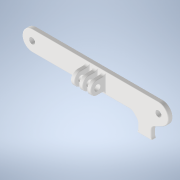
# Autodesk Inventor part: BackPlate
Saved by Autodesk Inventor 2021.3 (Build 253353010, 353A)
## iProperties
Created: 2021-08-11
Part Number: BackPlate
Material: Generisch
Document SubType Name: Modeling
Designer: Markus
Density: 1 g/cm^3
Appearance: Vorgabe
Author: Markus
Autodesk Inventor part; units mm, degrees
ref_plane "YZ Plane" through (0, 0, 0) normal (1, 0, 0) x (0, 1, 0)
ref_plane "XZ Plane" through (0, 0, 0) normal (0, 1, 0) x (-1, 0, 0)
ref_plane "XY Plane" through (0, 0, 0) normal (0, 0, 1) x (1, 0, 0)
sketch "Skizze2" plane through (0, 0, 0) normal (0, 0, 1) x (1, 0, 0)
  circle A0 centre (-47.5, 0) radius 2.408 projected
  spline S0 degree 3 poles (49.5, 0) (49.4999, -0.2484) (49.4548, -0.5089) (49.2125, -1.0889) (49.0309, -1.2975) (48.7582, -1.5703) (48.5453, -1.731) (48.0037, -1.9569) (47.7467, -1.9965) (47.2909, -2.0034) (47.0244, -1.964) (46.487, -1.7487) (46.2786, -1.598) (45.965, -1.3008) (45.7973, -1.0919) (45.5661, -0.5741) (45.5068, -0.3132) (45.4951, 0.1837) (45.5289, 0.4397) (45.7314, 0.9792) (45.8833, 1.1989) (46.2267, 1.567) (46.4444, 1.7165) (46.9007, 1.9251) (47.1526, 1.9859) (47.6719, 2.0102) (47.9359, 1.9699) (48.426, 1.7911) (48.6459, 1.6588) (49.0294, 1.3148) (49.1871, 1.1055) (49.4158, 0.6317) (49.483, 0.3718) (49.5059, -0.0571) (49.5014, -0.3263) (49.3091, -0.8923) (49.1761, -1.1223) (48.7992, -1.5514) (48.5744, -1.7005) (48.1516, -1.9082) (47.9012, -1.9759) (47.379, -2.0142) (47.1127, -1.9802) (46.6164, -1.8125) (46.3915, -1.6845) (45.9998, -1.3478) (45.8386, -1.1432) (45.5989, -0.6757) (45.5252, -0.4144) (45.4889, 0.0756) (45.5077, 0.3319) (45.6649, 0.8307) (45.7859, 1.0688) (46.1745, 1.5312) (46.4014, 1.6839) (46.8129, 1.8958) (47.0618, 1.9681) (47.6036, 2.0179) (47.8688, 1.9805) (48.3226, 1.8379) (48.5568, 1.7213) (48.9882, 1.3646) (49.1468, 1.159) (49.3855, 0.718) (49.4651, 0.4586) (49.5149, -0.0583) (49.4916, -0.3114) (49.3754, -0.7146) (49.2791, -0.9773) (48.883, -1.4729) (48.6723, -1.6385) (48.2327, -1.8787) (47.986, -1.9568) (47.4539, -2.0188) (47.1942, -1.9917) (46.756, -1.8682) (46.5093, -1.7643) (46.0388, -1.3961) (45.8712, -1.1849) (45.6506, -0.7906) (45.5549, -0.5486) (45.4775, 0.0404) (45.5118, 0.3057) (45.6296, 0.7488) (45.7375, 0.9855) (46.0612, 1.4125) (46.2535, 1.5852) (46.7029, 1.8534) (46.9543, 1.9423) (47.5294, 2.0243) (47.7984, 1.9884) (48.2415, 1.8743) (48.471, 1.7665) (48.9025, 1.4534) (49.0822, 1.2491) (49.3309, 0.8369) (49.4293, 0.5973) (49.5203, 0.0353) (49.5003, -0.2264) (49.3956, -0.6801) (49.2956, -0.9278) (48.9765, -1.373) (48.7884, -1.5513) (48.3813, -1.8093) (48.1346, -1.921) (47.5473, -2.0204) (47.2807, -2.0017) (46.7822, -1.8871) (46.5512, -1.7754) (46.1433, -1.4937) (45.9552, -1.2978) (45.6737, -0.8552) (45.5789, -0.6134) (45.4861, -0.1049) (45.4894, 0.1543) (45.5958, 0.6669) (45.7007, 0.9133) (45.9974, 1.3444) (46.1823, 1.5263) (46.5664, 1.7805) (46.8093, 1.9037) (47.3804, 2.0136) (47.6462, 2.0118) (48.2049, 1.8967) (48.4387, 1.7768) (48.8257, 1.5214) (49.0177, 1.3295) (49.3097, 0.8904) (49.4097, 0.6486) (49.5112, 0.143) (49.5131, -0.1147) (49.4169, -0.6302) (49.3158, -0.8803) (49.0266, -1.3169) (48.8451, -1.5021) (48.4436, -1.7786) (48.2042, -1.8945) (47.6624, -2.0105) (47.3974, -2.0146) (46.8418, -1.9125) (46.6055, -1.8006) (46.2068, -1.5487) (46.0132, -1.3634) (45.6983, -0.9137) (45.6, -0.6683) (45.4987, -0.2146) (45.4809, 0.0417) (45.5679, 0.5809) (45.6616, 0.8311) (45.9276, 1.2587) (46.0988, 1.4525) (46.371, 1.6523) (46.4267, 1.6889) (46.5266, 1.7478) (46.5702, 1.7715) (46.6733, 1.8225) (46.7334, 1.8484) (46.8365, 1.8872) (46.8793, 1.9017) (46.9444, 1.9214) (46.9664, 1.9276) (46.9994, 1.9364) (47.0105, 1.9392) (47.0324, 1.9446) (47.0411, 1.9467) (47.055, 1.9499) knots -7.965563 -7.965563 -7.965563 -7.965563 -7.879878 -7.879878 -7.775933 -7.775933 -7.637096 -7.637096 -7.502303 -7.502303 -7.353289 -7.353289 -7.204313 -7.204313 -7.050891 -7.050891 -6.916528 -6.916528 -6.799787 -6.799787 -6.676821 -6.676821 -6.527582 -6.527582 -6.372473 -6.372473 -6.211341 -6.211341 -6.055863 -6.055863 -5.89713 -5.89713 -5.736133 -5.736133 -5.636646 -5.636646 -5.558136 -5.558136 -5.466551 -5.466551 -5.357138 -5.357138 -5.243045 -5.243045 -5.13302 -5.13302 -5.022453 -5.022453 -4.908273 -4.908273 -4.812824 -4.812824 -4.73083 -4.73083 -4.639185 -4.639185 -4.524818 -4.524818 -4.396814 -4.396814 -4.272633 -4.272633 -4.150707 -4.150707 -4.012003 -4.012003 -3.882134 -3.882134 -3.795246 -3.795246 -3.723503 -3.723503 -3.647638 -3.647638 -3.565157 -3.565157 -3.495008 -3.495008 -3.42854 -3.42854 -3.368826 -3.368826 -3.306751 -3.306751 -3.236245 -3.236245 -3.17149 -3.17149 -3.104728 -3.104728 -3.025673 -3.025673 -2.930316 -2.930316 -2.823096 -2.823096 -2.726193 -2.726193 -2.627121 -2.627121 -2.525192 -2.525192 -2.435262 -2.435262 -2.35659 -2.35659 -2.281415 -2.281415 -2.193498 -2.193498 -2.090417 -2.090417 -1.990838 -1.990838 -1.891283 -1.891283 -1.788434 -1.788434 -1.689604 -1.689604 -1.611023 -1.611023 -1.545671 -1.545671 -1.469561 -1.469561 -1.365272 -1.365272 -1.263913 -1.263913 -1.163903 -1.163903 -1.059543 -1.059543 -0.959854 -0.959854 -0.869763 -0.869763 -0.788481 -0.788481 -0.695826 -0.695826 -0.576354 -0.576354 -0.448226 -0.448226 -0.325928 -0.325928 -0.209919 -0.209919 -0.105155 -0.105155 -0.079207 -0.079207 -0.060274 -0.060274 -0.03511 -0.03511 -0.017578 -0.017578 -0.008738 -0.008738 -0.004303 -0.004303 -0.000001 -0.000001 -0.000001 -0.000001 projected
  arc A1 (53.1427, -9.7735) -> (53.1427, 9.7735) centre (47.5, 0) ccw projected
  line L0 (-47.5, 0) -> (47.5, 0) construction
  circle A2 centre (-47.5, 0) radius 2.25
  circle A3 centre (47.5, 0) radius 2.25
  line L1 (42.01, -13.7) -> (42.01, -18)
  line L2 (42.01, -19) -> (32.01, -19)
  line L3 (32.01, -18) -> (32.01, -13.7)
  line L4 (32.29, -13.7) -> (41.73, -13.7) projected
  line L5 (45.2896, -14.5) -> (-45.2896, -14.5) projected
  line L6 (32.01, -19.5) -> (42.01, -19.5) construction
  line L7 (32.01, -20) -> (42.01, -20)
  line L8 (42.01, -19) -> (32.01, -19)
  arc A4 (31.61, -19.2) -> (32.01, -20) centre (32.01, -19.5) ccw
  arc A5 (42.01, -20) -> (42.41, -19.2) centre (42.01, -19.5) ccw
  arc A6 (42.01, -18) -> (42.41, -19.2) centre (44.01, -18) ccw
  arc A7 (31.61, -19.2) -> (32.01, -18) centre (30.01, -18) ccw
  arc A8 (32.01, -13.7) -> (30.8384, -10.8716) centre (28.01, -13.7) ccw
  arc A9 (44.1798, -10.1433) -> (42.01, -13.7) centre (46.01, -13.7) ccw
  arc A10 (-47.5, 7.5) -> (-47.5, -7.5) centre (-47.5, 0) ccw
  arc A11 (50.9317, -6.6688) -> (47.5, 7.5) centre (47.5, 0) ccw
  line L9 (-47.5, 7.5) -> (47.5, 7.5)
  line L10 (44.1798, -10.1433) -> (50.9317, -6.6688)
  line L11 (-47.5, -7.5) -> (25.81, -7.5)
  arc A12 (28.6384, -8.6716) -> (25.81, -7.5) centre (25.81, -11.5) ccw
  line L12 (28.6384, -8.6716) -> (30.8384, -10.8716)
  point P0 (0, 0)
  point P1 (0, 0)
  point P2 (37.01, -13.7)
  point P3 (37.01, -19)
  point P4 (37.01, -19.5)
  point P5 (37.01, -19)
  dimension "d3" = 4.5
  dimension "d4" = 4.5
  dimension "d28" = 10
  dimension "d29" = 4.5
  dimension "d30" = 1
  dimension "d48" = 2
  dimension "d49" = 4
  dimension "d54" = 15
  dimension "d55" = 4
  dimension "d59" = 135
  constraints: 26 end point, 20 point on circle, 19 tangent, 11 centre point, 6 vertical alignment, 5 midpoint, 4 horizontal, 4 point on line, 2 coincident, 2 concentric, 2 equal radius, 2 horizontal alignment, 2 parallel
  measures "d3" diameter of A2
  measures "d4" diameter of A3
  measures "d28" distance of L2.start L2.end
  measures "d29" distance between parallel lines of L5 L2
  measures "d30" distance between parallel lines of L7 L2
  measures "d48" radius of A6
  measures "d49" radius of A8
  measures "d54" distance between parallel lines of L9 L11
  measures "d55" radius of A12
  measures "d59" angle of L11 L12
extrude "Extrusion1" add sketch "Skizze2" along normal blind 3 contours A0 | L1 L5 L3 A8 L12 A12 L11 A10 L9 A11 L10 A9 | L1 A6 A5 L7 A4 A7 L3 L5
sketch "Skizze3" plane through (0, 0, 3) normal (0, 0, 1) x (1, 0, 0)
  line L0 (1.5, -5) -> (-1.5, -5)
  line L1 (-1.5, -5) -> (-1.5, 5)
  line L2 (-1.5, 5) -> (1.5, 5)
  line L3 (1.5, 5) -> (1.5, -5)
  line L4 (7.57, -5) -> (4.57, -5)
  line L5 (4.57, -5) -> (4.57, 5)
  line L6 (4.57, 5) -> (7.57, 5)
  line L7 (7.57, 5) -> (7.57, -5)
  line L8 (-4.57, -5) -> (-7.57, -5)
  line L9 (-7.57, -5) -> (-7.57, 5)
  line L10 (-7.57, 5) -> (-4.57, 5)
  line L11 (-4.57, 5) -> (-4.57, -5)
  point P0 (0, 0)
  point P1 (-1.5, 0)
  point P2 (0, -5)
  point P3 (6.07, -5)
  point P4 (4.57, 0)
  point P5 (-6.07, -5)
  point P6 (-7.57, 0)
  dimension "d7" = 10
  dimension "d8" = 3
  dimension "d11" = 6.07
  dimension "d18" = 6.07
  constraints: 24 end point, 3 horizontal, 2 collinear, 2 midpoint, 2 parallel, 1 horizontal alignment, 1 perpendicular, 1 vertical alignment, 18 other
  measures "d7" distance of L0.end L1.end
  measures "d8" distance of L1.end L2.end
  measures "d11" distance of L0.start L4.start
  measures "d18" distance of L0.start L8.start
extrude "Extrusion2" add sketch "Skizze3" along normal blind 11
sketch "Skizze4" plane through (-7.57, -5, 3) normal (-1, 0, 0) x (0, 0, 1)
  line L0 (0, 0) -> (0, 10) projected
  line L1 (0, 0) -> (11, 0) projected
  line L2 (11, 10) -> (11, 0) projected
  line L3 (0, 10) -> (11, 10) projected
  line L4 (0, 0) -> (11, 0) projected
  arc A0 (6, 0) -> (6, 10) centre (6, 5) ccw
  line L5 (6, 0) -> (0, 0)
  line L6 (0, 10) -> (11, 10) projected
  line L7 (6, 10) -> (0, 10)
  circle A1 centre (6, 5) radius 2.25
  point P0 (-3, 5)
  point P1 (11, 5)
  dimension "d25" = 4.5
  constraints: 4 end point, 3 tangent, 2 centre point, 2 point on circle, 2 point on line, 1 coincident, 1 collinear, 1 horizontal
  measures "d25" diameter of A1
extrude "Extrusion3" cut sketch "Skizze4" against normal through all contours A0 L2 L1 | L3 L2 A0 | A1
fillet "Rundung1" radius 2 6 edges at (-6.07, 5, 3) (0, 5, 3) (6.07, 5, 3) (-6.07, -5, 3) (0, -5, 3) (6.07, -5, 3)
fillet "Rundung1" radius 0.5 6 edges at (4.57, 0, 3) (7.57, 0, 3) (-1.5, 0, 3) (1.5, 0, 3) (-7.57, 0, 3) (-4.57, 0, 3)
fillet "Rundung3" radius 0.5 42 edges at (-4.57, 0, 14) (-4.57, 5, 7) (-4.57, 5.1771, 4.1771) (-4.4009, 6.3036, 3.1251) (-4.57, -5.1771, 4.1771) (-4.4009, -6.3036, 3.1251) (-4.57, -5, 7) (-7.57, 0, 14) (-7.57, 5, 7) (-7.57, 5.1771, 4.1771) (-7.7391, 6.3036, 3.1251) (-7.57, -5.1771, 4.1771) (-7.7391, -6.3036, 3.1251) (-7.57, -5, 7) (-1.5, 5, 7) (-1.5, 5.1771, 4.1771) (-1.6691, 6.3036, 3.1251) (-1.5, -5, 7) (-1.5, -5.1771, 4.1771) (-1.6691, -6.3036, 3.1251) (-1.5, 0, 14) (1.5, -5, 7) (1.5, -5.1771, 4.1771) (1.6691, -6.3036, 3.1251) (1.5, 5, 7) (1.5, 5.1771, 4.1771) (1.6691, 6.3036, 3.1251) (1.5, 0, 14) (4.57, 5, 7) (4.57, 5.1771, 4.1771) (4.4009, 6.3036, 3.1251) (4.57, -5, 7) (4.57, -5.1771, 4.1771) (4.4009, -6.3036, 3.1251) (4.57, 0, 14) (7.57, -5, 7) (7.57, -5.1771, 4.1771) (7.7391, -6.3036, 3.1251) (7.57, 5, 7) (7.57, 5.1771, 4.1771) (7.7391, 6.3036, 3.1251) (7.57, 0, 14)
fillet "Rundung4" radius 0.5 16 edges at (42.5953, -11.6168, 3) (47.5557, -8.4061, 3) (54.7893, 1.7655, 3) (0, 7.5, 3) (-55, 0, 3) (-10.845, -7.5, 3) (27.3407, -7.8045, 3) (29.7384, -9.7716, 3) (31.7055, -12.1693, 3) (32.01, -15.85, 3) (31.9074, -18.6325, 3) (31.5628, -19.7236, 3) (37.01, -20, 3) (42.4572, -19.7236, 3) (42.1126, -18.6325, 3) (42.01, -15.85, 3)
equation "\"d4\" = d3"
equation "\"d11\" = d18"
